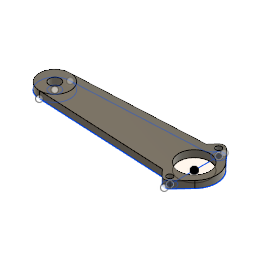
Arm v1 (Autodesk Fusion 360 design; units mm, degrees)
Autodesk Fusion 360 part; units mm, degrees
sketch "Sketch1" plane through (0, 0, 0) normal (0, 1, 0) x (1, 0, 0)
  circle A0 centre (0, 0) radius 11.05
  circle A1 centre (-100, 0) radius 11.05
  line L0 (-100, -11.05) -> (-7.1841, -15.6627)
  line L1 (0, 0) -> (0, 17.5)
  circle A2 centre (0, 17.5) radius 2.1
  circle A3 centre (0, 17.5) radius 4
  line L2 (0, 0) -> (0, -17.5)
  circle A4 centre (0, -17.5) radius 2.1
  circle A5 centre (0, -17.5) radius 4
  line L3 (0, -17.5) -> (0, -21.5)
  line L4 (11.5454, -11.0772) -> (2.9116, -20.2427)
  line L5 (0, 17.5) -> (0, 21.5)
  line L6 (11.5454, 11.0772) -> (2.9116, 20.2427)
  line L7 (-7.1841, -15.6627) -> (-2.9249, -20.2285)
  line L8 (-7.1841, 15.6627) -> (-2.9249, 20.2285)
  line L9 (-100, 11.05) -> (-7.1841, 15.6627)
  arc A6 (11.5454, -11.0772) -> (11.5454, 11.0772) centre (0, 0) ccw
  circle A7 centre (-100, 0) radius 4
  dimension "d1" = 22.1
  dimension "d2" = 22.1
  dimension "d8" = 17.5
  dimension "d9" = 4.2
  dimension "d10" = 8
  dimension "d11" = 17.5
  dimension "d12" = 4.2
  dimension "d13" = 8
  dimension "d16" = 8
  measures "d1" diameter of A0
  measures "d2" diameter of A1
  measures "d8" distance of A0.centre
  measures "d9" diameter of A2
  measures "d10" diameter of A3
  measures "d11" distance of A0.centre
  measures "d12" diameter of A4
  measures "d13" diameter of A5
  measures "d16" diameter of A7
extrude "Extrude2" add sketch "Sketch1" along normal blind 5 contours A0 L1 A3 L2 A5 L4 L6 A6 | A0 A1 L0 L1 A3 L2 A5 L7 L8 L9 | L1 A2 A3 L5 | L1 A2 A3 L5 | L2 A4 A5 L3 | L2 A4 A5 L3 | A1 | A7 makes body 1
extrude "Extrude1" add sketch "Sketch1" along normal blind 5 separate body contours A1 | A7 makes body 2
extrude "Extrude3" cut sketch "Sketch1" along normal blind 6 contours A7 bodies 1 2
